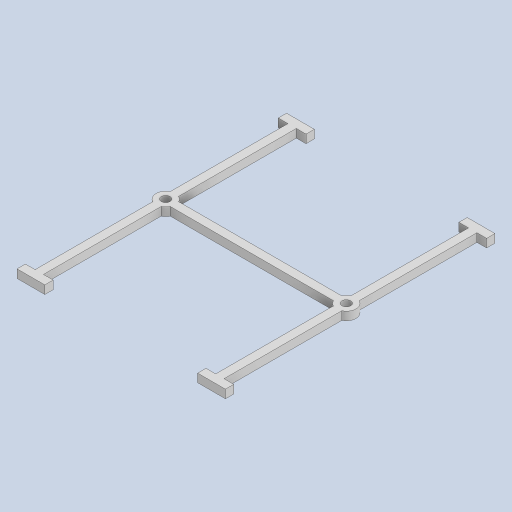
# Autodesk Inventor part: RSP-Spacer
Saved by Autodesk Inventor 2023.2 (Build 272271000, 271)
## iProperties
Created: 2024-03-26
Part Number: RSP-Spacer
Material: Generisch
Document SubType Name: Modeling
Designer: Nils Bade
Density: 1 g/cm^3
Appearance: Vorgabe
Author: Nils Bade
Autodesk Inventor part; units mm, degrees
ref_plane "YZ Plane" through (0, 0, 0) normal (1, 0, 0) x (0, 1, 0)
ref_plane "XZ Plane" through (0, 0, 0) normal (0, 1, 0) x (-1, 0, 0)
ref_plane "XY Plane" through (0, 0, 0) normal (0, 0, 1) x (1, 0, 0)
sketch "Skizze1" plane through (0, 0, 0) normal (0, 1, 0) x (-1, 0, 0)
  circle A0 centre (0, 0) radius 1.6
  circle A1 centre (0, 0) radius 3.5
  line L0 (-1.5, 3.1623) -> (-1.5, 48.5)
  line L1 (-1.5, 48.5) -> (1.5, 48.5)
  line L2 (1.5, 48.5) -> (1.5, 3.1623)
  line L3 (0, -67.9) -> (0, 67.9) construction
  line L4 (-40, 0) -> (12.5, 0) construction
  line L5 (-5, 45.5) -> (5, 45.5)
  line L6 (5, 45.5) -> (5, 48.5)
  line L7 (5, 48.5) -> (-5, 48.5)
  line L8 (-5, 48.5) -> (-5, 45.5)
  line L9 (-5, 45.5) -> (5, 48.5) construction
  line L10 (5, 45.5) -> (-5, 48.5) construction
  line L11 (-1.5, -3.1623) -> (-1.5, -48.5)
  line L12 (-1.5, -48.5) -> (1.5, -48.5)
  line L13 (1.5, -48.5) -> (1.5, -3.1623)
  line L14 (-5, -45.5) -> (5, -45.5)
  line L15 (5, -45.5) -> (5, -48.5)
  line L16 (5, -48.5) -> (-5, -48.5)
  line L17 (-5, -48.5) -> (-5, -45.5)
  line L18 (-5, -45.5) -> (5, -48.5) construction
  line L19 (5, -45.5) -> (-5, -48.5) construction
  line L20 (-3.1623, 1.5) -> (-32.5, 1.5)
  line L21 (-32.5, 1.5) -> (-32.5, -1.5)
  line L22 (-32.5, -1.5) -> (-3.1623, -1.5)
  line L23 (-3.1623, -1.5) -> (-3.1623, 1.5)
  point P0 (0, 47)
  point P1 (0, -47)
  point P2 (-3.1623, -1.5)
  point P3 (-1.5, -45.5)
  point P4 (1.5, -45.5)
  point P5 (1.5, -3.1623)
  point P6 (1.5, 45.5)
  point P7 (-1.5, 45.5)
  dimension "d0" = 3.2
  dimension "d1" = 7
  dimension "d2" = 3
  dimension "d3" = 48.5
  dimension "d4" = 3
  dimension "d5" = 10
  dimension "d6" = 3
  dimension "d7" = 32.5
  constraints: 44 end point, 9 symmetric about line, 5 parallel, 4 midpoint, 3 perpendicular, 2 centre point, 2 coincident, 2 point on circle, 1 collinear, 1 horizontal, 1 point on line, 2 other
  measures "d0" diameter of A0
  measures "d1" diameter of A1
  measures "d2" distance between parallel lines of L0 L2
  measures "d3" distance between parallel lines of L1 L4
  measures "d4" distance between parallel lines of L7 L5
  measures "d5" distance of L6.end L7.end
  measures "d6" distance between parallel lines of L20 L22
  measures "d7" distance between parallel lines of L21 L3
extrude "Extrusion1" add sketch "Skizze1" along normal blind 3
mirror "Spiegeln1" about plane through (32.5, 0, 1.5) normal (1, 0, 0)
